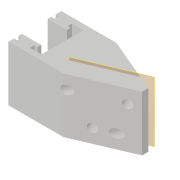
# Autodesk Inventor part: XRailSplitter
Saved by Autodesk Inventor 2018 (Build 220112000, 112)
## iProperties
Created: 2019-04-10
Part Number: XRailSplitter
Material: Generic
Document SubType Name: Modeling
Designer: ball
Density: 1 g/cm^3
Appearance: Default
Author: ball
Autodesk Inventor part; units mm, degrees
ref_plane "YZ Plane" through (0, 0, 0) normal (1, 0, 0) x (0, 1, 0)
ref_plane "XZ Plane" through (0, 0, 0) normal (0, 1, 0) x (-1, 0, 0)
ref_plane "XY Plane" through (0, 0, 0) normal (0, 0, 1) x (1, 0, 0)
sketch "Sketch1" plane through (0, 0, 0) normal (0, 1, 0) x (-1, 0, 0)
  line L0 (0, 0) -> (-12.7, 0)
  line L1 (-12.7, 0) -> (-12.7, -2.54)
  line L2 (-12.7, -2.54) -> (0, -2.54)
  line L3 (0, -2.54) -> (0, 0)
  line L4 (0, -21.844) -> (-12.7, -21.844)
  line L5 (-12.7, -21.844) -> (-12.7, -24.384)
  line L6 (-12.7, -24.384) -> (0, -24.384)
  line L7 (0, -24.384) -> (0, -21.844)
  line L8 (-12.7, 0) -> (-25.4, 0)
  line L9 (-25.4, 0) -> (-25.4, -24.384)
  line L10 (-25.4, -24.384) -> (-12.7, -24.384)
  line L11 (-12.7, -24.384) -> (-12.7, 0)
  line L12 (-25.4, 0) -> (-50.8, -10.7817)
  line L13 (-25.4, 0) -> (2.1936, 0) construction
  line L14 (-25.4, -24.384) -> (-50.8, -13.6023)
  line L15 (-25.4, -24.384) -> (2.1936, -24.384) construction
  line L16 (-50.8, -10.7817) -> (-50.8, -13.6023)
  line L17 (-1.4478, -4.572) -> (-7.4422, -4.572)
  line L18 (-7.4422, -4.572) -> (-7.4422, -2.54)
  line L19 (-7.4422, -2.54) -> (-1.4478, -2.54)
  line L20 (-1.4478, -2.54) -> (-1.4478, -4.572)
  line L21 (-1.4478, -21.844) -> (-7.4422, -21.844)
  line L22 (-7.4422, -21.844) -> (-7.4422, -19.812)
  line L23 (-7.4422, -19.812) -> (-1.4478, -19.812)
  line L24 (-1.4478, -19.812) -> (-1.4478, -21.844)
  line L25 (0, -19.812) -> (-8.89, -19.812)
  line L26 (-8.89, -19.812) -> (-8.89, -18.161)
  line L27 (-8.89, -18.161) -> (0, -18.161)
  line L28 (0, -18.161) -> (0, -19.812)
  line L29 (0, -4.572) -> (-8.89, -4.572)
  line L30 (-8.89, -4.572) -> (-8.89, -6.223)
  line L31 (-8.89, -6.223) -> (0, -6.223)
  line L32 (0, -6.223) -> (0, -4.572)
  dimension "d2" = 12.7
  dimension "d3" = 2.54
  dimension "d4" = 12.7
  dimension "d5" = 2.54
  dimension "d6" = 24.384
  dimension "d7" = 12.7
  dimension "d8" = 24.384
  dimension "d9" = 157
  dimension "d10" = 157
  dimension "d11" = 25.4
  dimension "d12" = 25.4
  dimension "d15" = 5.9944
  dimension "d16" = 2.032
  dimension "d17" = 2.032
  dimension "d18" = 1.4478
  dimension "d19" = 5.9944
  dimension "d20" = 2.032
  dimension "d21" = 1.4478
  dimension "d22" = 8.89
  dimension "d23" = 1.651
  dimension "d24" = 8.89
  dimension "d25" = 1.651
  constraints: 66 end point, 14 parallel, 9 horizontal, 7 perpendicular, 2 equal length, 2 point on line
  measures "d2" distance of L2.end L1.end
  measures "d3" distance of L1.end L0.end
  measures "d4" distance of L6.end L5.end
  measures "d5" distance of L5.end L4.end
  measures "d6" distance between parallel lines of L6 L0
  measures "d7" distance of L10.end L9.end
  measures "d8" distance of L9.end L8.end
  measures "d9" angle of L12 L13
  measures "d10" angle of L15 L14
  measures "d11" distance from line of L12.end L9
  measures "d12" distance from line of L14.end L9
  measures "d15" distance of L18.end L19.end
  measures "d16" distance of L17.end L18.end
  measures "d17" distance between parallel lines of L17 L2
  measures "d18" distance between parallel lines of L3 L20
  measures "d19" distance of L22.end L23.end
  measures "d20" distance of L21.end L22.end
  measures "d21" distance between parallel lines of L24 L7
  measures "d22" distance of L26.end L27.end
  measures "d23" distance of L25.end L26.end
  measures "d24" distance of L31.end L30.end
  measures "d25" distance of L30.end L29.end
extrude "Extrusion1" add sketch "Sketch1" along normal blind 25.4
sketch "Sketch2" plane through (25.4, 0, -24.384) normal (0.3907, 0, -0.9205) x (-0.9205, 0, -0.3907)
  circle A0 centre (-10.16, 19.05) radius 1.9685
  circle A1 centre (-22.5136, 6.35) radius 1.9685
  line L0 (-27.5936, 0) -> (0, 0) projected
  line L1 (-27.5936, 0) -> (-27.5936, 25.4) projected
  line L2 (0, 0) -> (0, 25.4) projected
  line L3 (-27.5936, 25.4) -> (0, 25.4) projected
  point P0 (13.8532, 0)
  dimension "d28" = 3.937
  dimension "d29" = 3.937
  dimension "d30" = 6.35
  dimension "d31" = 5.08
  dimension "d32" = 10.16
  dimension "d33" = 6.35
  constraints: 2 centre point
  measures "d28" diameter of A0
  measures "d29" diameter of A1
  measures "d30" distance from line of L0 A1.centre
  measures "d31" distance from line of L1 A1.centre
  measures "d32" distance from line of L2 A0.centre
  measures "d33" distance from line of L3 A0.centre
hole "Hole1" at (34.7523, 19.05, -20.4142) at (46.1238, 6.35, -15.5873) direction (-0.3907, 0, 0.9205) diameter 3.937 end through all
sketch "Sketch3" plane through (50.8, 0, -10.7817) normal (0.3907, 0, 0.9205) x (0.9205, 0, -0.3907)
  circle A0 centre (-5.08, 19.05) radius 1.9685
  circle A1 centre (-17.4336, 6.35) radius 1.9685
  line L0 (-27.5936, 25.4) -> (0, 25.4) projected
  line L1 (0, 0) -> (0, 25.4) projected
  line L2 (-27.5936, 0) -> (0, 0) projected
  line L3 (-27.5936, 0) -> (-27.5936, 17.1859) projected
  point P0 (-50.9744, 0)
  dimension "d41" = 3.937
  dimension "d42" = 3.937
  dimension "d43" = 6.35
  dimension "d44" = 5.08
  dimension "d45" = 6.35
  dimension "d46" = 10.16
  constraints: 2 centre point
  measures "d41" diameter of A0
  measures "d42" diameter of A1
  measures "d43" distance from line of L0 A0.centre
  measures "d44" distance from line of L1 A0.centre
  measures "d45" distance from line of L2 A1.centre
  measures "d46" distance from line of L3 A1.centre
hole "Hole2" at (46.1238, 19.05, -8.7967) at (34.7523, 6.35, -3.9698) direction (-0.3907, 0, -0.9205) diameter 3.937 end through all
ref_plane "Work Plane1" through (47.8226, 0, -17.7959) normal (0.3907, 0, 0.9205) x (0.9205, 0, -0.3907)
body "Solid1"
